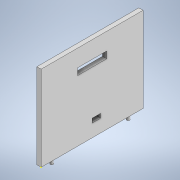
# Autodesk Inventor part: expo3
Saved by Autodesk Inventor 2020 (Build 240168000, 168)
## iProperties
Created: 2020-02-18
Part Number: expo3
Material: Generic
Document SubType Name: Modeling
Designer: Aryan
Density: 1 g/cm^3
Appearance: Default
Author: Aryan
Autodesk Inventor part; units mm, degrees
ref_plane "YZ Plane" through (0, 0, 0) normal (1, 0, 0) x (0, 1, 0)
ref_plane "XZ Plane" through (0, 0, 0) normal (0, 1, 0) x (-1, 0, 0)
ref_plane "XY Plane" through (0, 0, 0) normal (0, 0, 1) x (1, 0, 0)
sketch "Sketch1" plane through (0, 0, 0) normal (0, 1, 0) x (-1, 0, 0)
  line L0 (0, 0) -> (-5, 0)
  line L1 (-5, 0) -> (-5, -120)
  line L2 (-5, -120) -> (0, -120)
  line L3 (0, -120) -> (0, 0)
  dimension "d0" = 5
  dimension "d1" = 120
  constraints: 8 end point, 2 parallel, 1 horizontal, 1 perpendicular
  measures "d0" distance of L2.end L1.end
  measures "d1" distance of L1.end L0.end
extrude "Extrusion1" add sketch "Sketch1" along normal blind 100
sketch "Sketch2" plane through (0, 0, 0) normal (0, -1, 0) x (1, 0, 0)
  line L0 (0, -120) -> (0, 0) projected
  line L1 (0, 0) -> (2.5, 0)
  line L2 (2.5, 0) -> (2.5, -15)
  line L3 (2.5, -15) -> (0, -15)
  line L4 (0, -15) -> (0, 0)
  circle A0 centre (2.5, -15) radius 1.75
  dimension "d4" = 2.5
  dimension "d5" = 15
  dimension "d6" = 3.5
  constraints: 8 end point, 2 parallel, 1 centre point, 1 coincident, 1 horizontal, 1 perpendicular
  measures "d4" distance of L2.end L3.end
  measures "d5" distance of L1.end L2.end
  measures "d6" diameter of A0
extrude "Extrusion2" add sketch "Sketch2" along normal blind 5 contours A0 L2 L3 | L3 L2 A0
sketch "Sketch3" plane through (0, 0, 0) normal (0, -1, 0) x (1, 0, 0)
  line L0 (5, 0) -> (5, -120) projected
  line L1 (5, -120) -> (2.5, -120)
  line L2 (2.5, -120) -> (2.5, -105)
  line L3 (2.5, -105) -> (5, -105)
  line L4 (5, -105) -> (5, -120)
  circle A0 centre (2.5, -105) radius 1.75
  point P0 (0, 0)
  dimension "d9" = 2.5
  dimension "d10" = 15
  dimension "d11" = 3.5
  constraints: 8 end point, 2 parallel, 1 centre point, 1 coincident, 1 horizontal, 1 perpendicular
  measures "d9" distance of L2.end L3.end
  measures "d10" distance of L1.end L2.end
  measures "d11" diameter of A0
extrude "Extrusion3" add sketch "Sketch3" along normal blind 5 contours A0 L2 L3 | L3 L2 A0
sketch "Sketch4" plane through (5, 0, 0) normal (1, 0, 0) x (0, 0, -1)
  point P0 (0, 0)
sketch "Sketch5" plane through (5, 0, 0) normal (1, 0, 0) x (0, 0, -1)
  point P0 (0, 0)
sketch "Sketch6" plane through (5, 0, 0) normal (1, 0, 0) x (0, 0, -1)
  point P0 (0, 0)
sketch "Sketch7" plane through (5, 0, 0) normal (1, 0, 0) x (0, 0, -1)
  line L0 (120, 100) -> (0, 100) projected
  line L1 (0, 100) -> (42.838, 100)
  line L2 (42.838, 100) -> (42.838, 80)
  line L3 (42.838, 80) -> (0, 80)
  line L4 (0, 80) -> (0, 100)
  line L5 (42.838, 80) -> (77.174, 80)
  line L6 (77.174, 80) -> (77.174, 72)
  line L7 (77.174, 72) -> (42.838, 72)
  line L8 (42.838, 72) -> (42.838, 80)
  point P0 (0, 0)
  dimension "d14" = 42.838
  dimension "d15" = 20
  dimension "d16" = 34.336
  dimension "d17" = 8
  constraints: 16 end point, 4 parallel, 2 horizontal, 2 perpendicular
  measures "d14" distance of L2.end L3.end
  measures "d15" distance of L1.end L2.end
  measures "d16" distance of L6.end L7.end
  measures "d17" distance of L5.end L6.end
extrude "Extrusion4" cut sketch "Sketch7" against normal blind 10 contours L5 L6 L7 L8
sketch "Sketch8" plane through (5, 0, 0) normal (1, 0, 0) x (0, 0, -1)
  line L0 (0, 0) -> (60, 0)
  line L1 (60, 0) -> (60, 15)
  line L2 (60, 15) -> (0, 15)
  line L3 (0, 15) -> (0, 0)
  line L4 (60, 15) -> (70, 15)
  line L5 (70, 15) -> (70, 20)
  line L6 (70, 20) -> (60, 20)
  line L7 (60, 20) -> (60, 15)
  dimension "d20" = 60
  dimension "d21" = 15
  dimension "d22" = 10
  dimension "d23" = 5
  constraints: 16 end point, 4 parallel, 2 horizontal, 2 perpendicular
  measures "d20" distance of L2.end L1.end
  measures "d21" distance of L1.end L0.end
  measures "d22" distance of L6.end L5.end
  measures "d23" distance of L5.end L4.end
extrude "Extrusion5" cut sketch "Sketch8" against normal blind 10 contours L7 L6 L5 L4
body "Solid1"
